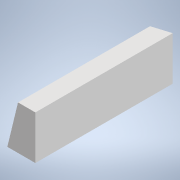
# Autodesk Inventor part: FrontBumperFillA
Saved by Autodesk Inventor 2020 (Build 240168000, 168)
## iProperties
Created: 2020-01-19
Part Number: FrontBumperFillA
Material: Generic
Document SubType Name: Modeling
Designer: srini
Density: 1 g/cm^3
Appearance: Default
Author: srini
Autodesk Inventor part; units mm, degrees
ref_plane "YZ Plane" through (0, 0, 0) normal (1, 0, 0) x (0, 1, 0)
ref_plane "XZ Plane" through (0, 0, 0) normal (0, 1, 0) x (-1, 0, 0)
sketch "Sketch1" plane through (0, 0, 0) normal (0, 0, 1) x (1, 0, 0)
  line L0 (-812.8, -3.937) -> (0, -3.937) projected
  line L1 (-30.988, 74.295) -> (-15.2847, 74.295) projected
  line L2 (0, -3.937) -> (-50.038, -3.937)
  line L3 (-50.038, -3.937) -> (-30.988, 74.295)
  line L4 (-30.988, 74.295) -> (0, 74.295)
  line L5 (0, 74.295) -> (0, -3.937)
  line L6 (-50.038, -7.112) -> (-50.038, -3.937) projected
  point P0 (0, 0)
  constraints: 8 end point, 3 point on line, 2 collinear, 1 horizontal, 1 parallel, 1 vertical
ref_plane "Work Plane1" through (-8.9942, -7.112, -242.5521) normal (-0.2905, 0, -0.9569) x (0, 1, 0)
extrude "Extrusion1" add sketch "Sketch1" against normal up to surface surface through (-8.9942, -7.112, -242.5521) normal (-0.2905, 0, -0.9569)
body "Solid1"
